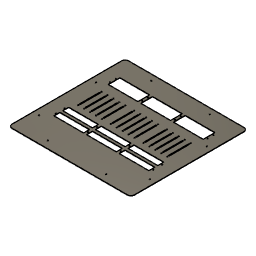
frontplate (Autodesk Fusion 360 design; units mm, degrees)
Autodesk Fusion 360 part; units mm, degrees
note: some values were not read from the file. Set by a fixed rule: which sketch regions a step uses.
sketch "Skizze1" plane through (0, 0, 0) normal (0, 1, 0) x (1, 0, 0)
  line L0 (198, -200) -> (-198, -200)
  line L1 (-210, -188) -> (-210, 188)
  line L2 (-198, 200) -> (198, 200)
  line L3 (210, 188) -> (210, -188)
  line L4 (210, -200) -> (-210, 200) construction
  line L5 (-210, -200) -> (210, 200) construction
  arc A0 (-198, 200) -> (-210, 188) centre (-198, 188) ccw
  arc A1 (210, 188) -> (198, 200) centre (198, 188) ccw
  arc A2 (198, -200) -> (210, -188) centre (198, -188) ccw
  arc A3 (-210, -188) -> (-198, -200) centre (-198, -188) ccw
  dimension "d1" = 420
  dimension "d2" = 400
  dimension "d3" = 12
  constraint perpendicular L0 L1
  constraint parallel L0 L2
  constraint parallel L1 L3
  constraint horizontal L0
  constraint coincident L4 origin
  constraint coincident L5 origin
  constraint coincident L4.end L1
  constraint coincident L4.end L2
  constraint tangent L1 A0
  constraint tangent L2 A0
  constraint coincident L5.end L2
  constraint coincident L5.end L3
  constraint tangent L2 A1
  constraint tangent L3 A1
  constraint equal A0 A1
  constraint coincident L4.start L3
  constraint coincident L4.start L0
  constraint tangent L3 A2
  constraint tangent L0 A2
  constraint equal A0 A2
  constraint coincident L5.start L1
  constraint coincident L5.start L0
  constraint tangent L1 A3
  constraint tangent L0 A3
  constraint equal A0 A3
  measures "d1" distance of L4.end L5.end
  measures "d2" distance of L5.start L4.end
  measures "d3" radius of A0
extrude "Fläche1" add sketch "Skizze1" along normal blind 1.5
sketch "Skizze2" plane through (0, 1.5, 0) normal (0, 1, 0) x (-1, 0, 0)
  arc A0 (198, -200) -> (210, -188) centre (198, -188) ccw
  line L0 (210, -188) -> (210, 188)
  arc A1 (210, 188) -> (198, 200) centre (198, 188) ccw
  line L1 (198, 200) -> (-198, 200)
  arc A2 (-198, 200) -> (-210, 188) centre (-198, 188) ccw
  line L2 (-210, 188) -> (-210, -188)
  arc A3 (-210, -188) -> (-198, -200) centre (-198, -188) ccw
  line L3 (-198, -200) -> (198, -200)
  circle A4 centre (-91.6, -62) radius 1.6
  line L4 (0, -62) -> (0, -57)
  line L5 (-130.9, -57) -> (-133.9, -57)
  line L6 (0, -200) -> (0, 200)
  line L7 (-110.5, 13) -> (-110.5, -57)
  circle A5 centre (-71.2, -62) radius 1.6
  line L8 (-110.5, -57) -> (-113.5, -57)
  line L9 (1.5, 13) -> (1.5, -57)
  line L10 (-69.7, 13) -> (-69.7, -57)
  circle A6 centre (-20.4, -62) radius 1.6
  circle A7 centre (0, -62) radius 1.6
  line L11 (-42.3, -57) -> (-42.3, 13)
  line L12 (-1.5, -57) -> (-1.5, 13)
  line L13 (-21.9, -57) -> (-21.9, 13)
  line L14 (-113.5, -57) -> (-113.5, 13)
  line L15 (-151.3, 13) -> (-151.3, -57)
  line L16 (-18.9, 13) -> (-18.9, -57)
  line L17 (-39.3, -57) -> (-42.3, -57)
  line L18 (-151.3, -57) -> (-154.3, -57)
  circle A8 centre (-40.8, -62) radius 1.6
  line L19 (210, -188) -> (210, 188)
  circle A9 centre (-132.4, -62) radius 1.6
  line L20 (-198, -200) -> (198, -200)
  line L21 (-130.9, 13) -> (-130.9, -57)
  line L22 (-18.9, -57) -> (-21.9, -57)
  line L23 (-210, 188) -> (-210, -188)
  circle A10 centre (-112, -62) radius 1.6
  line L24 (-39.3, 13) -> (-39.3, -57)
  line L25 (0, -57) -> (0, -62)
  line L26 (-10.2, 70.9) -> (10.2, 91.3) construction
  line L27 (72.7, 13) -> (72.7, -57)
  circle A11 centre (-168, -105) radius 1.6
  line L28 (154.3, 13) -> (154.3, -57)
  line L29 (-10.2, -135) -> (-30.6, -95) construction
  line L30 (-10.2, 40.5) -> (-30.6, 60.9) construction
  line L31 (72.7, -57) -> (69.7, -57)
  line L32 (154.3, -57) -> (151.3, -57)
  line L33 (133.9, -57) -> (130.9, -57)
  line L34 (-8.6, -135) -> (-8.6, -97)
  circle A12 centre (-20.4, 18) radius 1.6
  line L35 (198, 200) -> (-198, 200)
  line L36 (81.4, -135) -> (101.8, -95) construction
  line L37 (69.7, -57) -> (69.7, 13)
  line L38 (-51.8, -97) -> (-51.8, -135)
  line L39 (113.5, -57) -> (110.5, -57)
  line L40 (10.2, -95) -> (-10.2, -95)
  line L41 (-101.8, -135) -> (-81.4, -135)
  line L42 (0, 18) -> (0, 13)
  line L43 (113.5, 13) -> (113.5, -57)
  line L44 (-81.4, -135) -> (-61, -95) construction
  line L45 (-30.6, 60.9) -> (-30.6, 40.5)
  line L46 (-122.2, -135) -> (-101.8, -95) construction
  circle A13 centre (56, -105) radius 1.6
  circle A14 centre (40.8, -62) radius 1.6
  line L47 (10.2, 70.9) -> (-10.2, 91.3) construction
  line L48 (101.8, -135) -> (81.4, -95) construction
  line L49 (42.3, 13) -> (42.3, -57)
  circle A15 centre (112, -62) radius 1.6
  line L50 (-163, -95) -> (-163, -135)
  line L51 (-31.4, 84) -> (-31.4, 66)
  line L52 (-8.6, 66) -> (-8.6, 84)
  line L53 (-10.2, 70.9) -> (-30.6, 91.3) construction
  line L54 (-101.8, -135) -> (-101.8, -95)
  line L55 (-122.2, -95) -> (-142.6, -95)
  circle A16 centre (20.4, -62) radius 1.6
  line L56 (11.8, -135) -> (11.8, -97)
  line L57 (-30.6, -135) -> (-51, -95) construction
  line L58 (-81.4, -95) -> (-101.8, -95)
  line L59 (29.8, -97) -> (29.8, -135)
  line L60 (-51, -125) -> (-61, -125)
  line L61 (-51, -135) -> (-30.6, -95) construction
  line L62 (61, -95) -> (61, -135)
  line L63 (-142.6, -95) -> (-163, -95)
  line L64 (-10.2, 70.9) -> (-10.2, 91.3)
  line L65 (-81.4, -135) -> (-81.4, -95)
  line L66 (30.6, -135) -> (10.2, -95) construction
  line L67 (-10.2, 60.9) -> (-30.6, 60.9)
  line L68 (81.4, 40.5) -> (81.4, 60.9)
  line L69 (-101.8, -135) -> (-122.2, -95) construction
  line L70 (-30.6, 70.9) -> (-10.2, 70.9)
  line L71 (-142.6, -135) -> (-142.6, -95)
  line L72 (-101.8, -135) -> (-81.4, -95) construction
  line L73 (30.6, -95) -> (30.6, -135)
  line L74 (-163, -135) -> (-142.6, -135)
  line L75 (133.9, 13) -> (133.9, -57)
  line L76 (-11, -97) -> (-11, -135)
  line L77 (10.2, -135) -> (30.6, -135)
  circle A17 centre (-56, -125) radius 1.6
  line L78 (81.4, -135) -> (101.8, -135)
  circle A18 centre (152.8, -62) radius 1.6
  circle A19 centre (71.2, -62) radius 1.6
  line L79 (61, 40.5) -> (81.4, 40.5)
  line L80 (-81.4, -135) -> (-61, -135)
  line L81 (-122.2, -135) -> (-101.8, -135)
  line L82 (-122.2, -135) -> (-122.2, -95)
  line L83 (-122.2, -95) -> (-122.2, -135)
  line L84 (-10.2, -135) -> (-10.2, -95)
  line L85 (-10.2, 40.5) -> (10.2, 60.9) construction
  line L86 (-10.2, 91.3) -> (-10.2, 70.9)
  line L87 (-61, -135) -> (-61, -95)
  line L88 (18.9, -57) -> (18.9, 13)
  line L89 (10.2, 60.9) -> (-10.2, 60.9)
  line L90 (-30.6, 70.9) -> (-10.2, 91.3) construction
  circle A20 centre (56, -125) radius 1.6
  line L91 (30.6, -135) -> (30.6, -95)
  circle A21 centre (0, 18) radius 1.6
  line L92 (42.3, -57) -> (39.3, -57)
  line L93 (30.6, -135) -> (51, -135)
  line L94 (-30.6, -135) -> (-10.2, -95) construction
  line L95 (-122.2, -135) -> (-142.6, -95) construction
  circle A22 centre (91.6, -62) radius 1.6
  line L96 (-30.6, 91.3) -> (-30.6, 70.9)
  line L97 (21.9, -57) -> (18.9, -57)
  line L98 (51, 40.5) -> (51, 60.9)
  line L99 (51, -135) -> (30.6, -95) construction
  line L100 (-51, -95) -> (-51, -135)
  line L101 (-49.4, -135) -> (-49.4, -97)
  line L102 (69.7, 13) -> (72.7, 13)
  line L103 (61, -105) -> (51, -105)
  line L104 (151.3, -57) -> (151.3, 13)
  line L105 (-10.2, -135) -> (10.2, -95) construction
  line L106 (-61, -135) -> (-81.4, -95) construction
  line L107 (39.3, -57) -> (39.3, 13)
  line L108 (101.8, 91.3) -> (81.4, 91.3)
  line L109 (-122.2, 70.9) -> (-122.2, 91.3)
  line L110 (-81.4, -135) -> (-101.8, -95) construction
  line L111 (-61, -95) -> (-81.4, -95)
  line L112 (61, -135) -> (81.4, -135)
  line L113 (-21.9, 13) -> (-18.9, 13)
  line L114 (-101.8, -95) -> (-101.8, -135)
  line L115 (-122.2, 70.9) -> (-101.8, 70.9)
  circle A23 centre (20.4, 18) radius 1.6
  line L116 (-10.2, 40.5) -> (-10.2, 60.9)
  line L117 (110.5, -57) -> (110.5, 13)
  line L118 (-30.6, 70.9) -> (-30.6, 91.3)
  line L119 (-11, 56) -> (-11, 38)
  line L120 (130.9, -57) -> (130.9, 13)
  line L121 (122.2, 91.3) -> (101.8, 91.3)
  line L122 (61, -125) -> (51, -125)
  line L123 (-142.6, -135) -> (-122.2, -95) construction
  line L124 (-101.8, 70.9) -> (-81.4, 70.9)
  line L125 (101.8, -95) -> (81.4, -95)
  line L126 (-30.6, -135) -> (-10.2, -135)
  line L127 (-122.2, 40.5) -> (-101.8, 40.5)
  line L128 (51, 91.3) -> (30.6, 91.3)
  line L129 (10.2, 40.5) -> (10.2, 60.9)
  line L130 (30.6, 60.9) -> (30.6, 40.5)
  line L131 (-51, -135) -> (-30.6, -135)
  line L132 (142.6, -135) -> (163, -135)
  line L133 (-10.2, 60.9) -> (-10.2, 40.5)
  line L134 (-122.2, 91.3) -> (-142.6, 91.3)
  line L135 (-10.2, 40.5) -> (10.2, 40.5)
  line L136 (-101.8, 40.5) -> (-81.4, 40.5)
  line L137 (-81.4, 40.5) -> (-101.8, 60.9) construction
  line L138 (61, 60.9) -> (61, 40.5)
  line L139 (-81.4, 91.3) -> (-101.8, 91.3)
  line L140 (30.6, 40.5) -> (10.2, 60.9) construction
  line L141 (11.8, 38) -> (11.8, 56)
  line L142 (142.6, -135) -> (122.2, -95) construction
  line L143 (-30.6, 40.5) -> (-10.2, 40.5)
  circle A24 centre (71.2, 18) radius 1.6
  circle A25 centre (166.5, -105) radius 1.6
  line L144 (-101.8, 60.9) -> (-122.2, 60.9)
  line L145 (-122.2, 70.9) -> (-101.8, 91.3) construction
  line L146 (101.8, -135) -> (101.8, -95)
  line L147 (-113.5, 13) -> (-110.5, 13)
  line L148 (-101.8, 91.3) -> (-122.2, 91.3)
  line L149 (-122.2, 60.9) -> (-122.2, 40.5)
  circle A26 centre (-56, 81.1) radius 1.6
  line L150 (81.4, 60.9) -> (61, 60.9)
  line L151 (61, 40.5) -> (81.4, 60.9) construction
  line L152 (-51.8, 56) -> (-51.8, 38)
  line L153 (163, -105) -> (166.5, -105)
  line L154 (-30.6, -95) -> (-30.6, -135)
  line L155 (30.6, 60.9) -> (10.2, 60.9)
  line L156 (-122.2, 91.3) -> (-122.2, 70.9)
  line L157 (10.2, -135) -> (-10.2, -95) construction
  line L158 (10.2, 40.5) -> (30.6, 60.9) construction
  line L159 (-11, 84) -> (-11, 66)
  line L160 (142.6, -95) -> (122.2, -95)
  line L161 (-101.8, 70.9) -> (-101.8, 91.3)
  line L162 (10.2, 60.9) -> (10.2, 40.5)
  line L163 (-51, 81.1) -> (-61, 81.1)
  line L164 (30.6, -95) -> (10.2, -95)
  line L165 (-142.6, 91.3) -> (-163, 91.3)
  line L166 (122.2, -95) -> (122.2, -135)
  line L167 (-122.2, 40.5) -> (-101.8, 60.9) construction
  line L168 (10.2, 40.5) -> (30.6, 40.5)
  line L169 (122.2, -135) -> (142.6, -95) construction
  line L170 (-93.1, 13) -> (-90.1, 13)
  circle A27 centre (40.8, 18) radius 1.6
  line L171 (163, -125) -> (166.5, -125)
  line L172 (122.2, -135) -> (101.8, -95) construction
  line L173 (-51, 50.7) -> (-61, 50.7)
  line L174 (-72.7, 13) -> (-69.7, 13)
  circle A28 centre (166.5, -125) radius 1.6
  arc A29 (-198, 200) -> (-210, 188) centre (-198, 188) ccw
  line L175 (-81.4, 70.9) -> (-61, 91.3) construction
  line L176 (-81.4, 40.5) -> (-61, 40.5)
  line L177 (122.2, -135) -> (142.6, -135)
  line L178 (163, -95) -> (142.6, -95)
  line L179 (-30.6, 60.9) -> (-51, 60.9)
  line L180 (-42.3, 13) -> (-39.3, 13)
  line L181 (-30.6, 40.5) -> (-51, 60.9) construction
  line L182 (101.8, -135) -> (122.2, -135)
  line L183 (101.8, -95) -> (101.8, -135)
  line L184 (142.6, -135) -> (163, -95) construction
  line L185 (-51, 40.5) -> (-30.6, 40.5)
  line L186 (61, 50.7) -> (51, 50.7)
  line L187 (163, -135) -> (142.6, -95) construction
  line L188 (-81.4, 70.9) -> (-101.8, 91.3) construction
  line L189 (30.6, 40.5) -> (30.6, 60.9)
  line L190 (-81.4, 70.9) -> (-61, 70.9)
  line L191 (-61, 70.9) -> (-81.4, 91.3) construction
  line L192 (163, 91.3) -> (142.6, 91.3)
  line L193 (-101.8, 70.9) -> (-81.4, 91.3) construction
  line L194 (-8.6, 38) -> (-8.6, 56)
  line L195 (81.4, -135) -> (81.4, -95)
  line L196 (-163, -135) -> (-142.6, -95) construction
  line L197 (-29, 38) -> (-29, 56)
  line L198 (-29, -135) -> (-29, -97)
  circle A30 centre (132.4, -62) radius 1.6
  line L199 (93.1, 13) -> (93.1, -57)
  line L200 (-1.5, 13) -> (1.5, 13)
  line L201 (-30.6, 40.5) -> (-30.6, 60.9)
  line L202 (-10.2, -135) -> (10.2, -135)
  line L203 (10.2, 40.5) -> (-10.2, 60.9) construction
  line L204 (-101.8, -95) -> (-122.2, -95)
  circle A31 centre (56, 50.7) radius 1.6
  line L205 (81.4, 60.9) -> (81.4, 40.5)
  line L206 (51, -95) -> (30.6, -95)
  line L207 (-51, -105) -> (-61, -105)
  line L208 (-142.6, -95) -> (-142.6, -135)
  line L209 (30.6, 40.5) -> (51, 40.5)
  line L210 (81.4, -95) -> (61, -95)
  line L211 (21.9, 13) -> (21.9, -57)
  line L212 (-31.4, 56) -> (-31.4, 38)
  line L213 (-101.8, 40.5) -> (-101.8, 60.9)
  line L214 (90.1, -57) -> (90.1, 13)
  line L215 (142.6, 91.3) -> (122.2, 91.3)
  line L216 (-101.8, 91.3) -> (-101.8, 70.9)
  line L217 (30.6, -135) -> (51, -95) construction
  line L218 (81.4, 40.5) -> (61, 60.9) construction
  line L219 (93.1, -57) -> (90.1, -57)
  line L220 (-142.6, -135) -> (-163, -95) construction
  circle A32 centre (-168, -125) radius 1.6
  line L221 (-101.8, 60.9) -> (-101.8, 40.5)
  line L222 (10.2, 91.3) -> (-10.2, 91.3)
  line L223 (-30.6, -95) -> (-51, -95)
  line L224 (30.6, 91.3) -> (10.2, 91.3)
  line L225 (61, -135) -> (81.4, -95) construction
  line L226 (51, 60.9) -> (30.6, 60.9)
  line L227 (81.4, -135) -> (61, -95) construction
  line L228 (-30.6, -135) -> (-30.6, -95)
  line L229 (-81.4, -95) -> (-81.4, -135)
  line L230 (-101.8, 40.5) -> (-81.4, 60.9) construction
  line L231 (-142.6, -135) -> (-122.2, -135)
  line L232 (51, -135) -> (51, -95)
  line L233 (30.6, 40.5) -> (51, 60.9) construction
  line L234 (81.4, 91.3) -> (61, 91.3)
  circle A33 centre (-112, 18) radius 1.6
  line L235 (-81.4, 60.9) -> (-101.8, 60.9)
  line L236 (29.8, 56) -> (29.8, 38)
  line L237 (-10.2, 91.3) -> (-30.6, 91.3)
  line L238 (9.4, 56) -> (9.4, 38)
  line L239 (122.2, -135) -> (122.2, -95)
  line L240 (10.2, -135) -> (30.6, -95) construction
  line L241 (-31.4, -97) -> (-31.4, -135)
  line L242 (-101.8, 70.9) -> (-122.2, 91.3) construction
  line L243 (9.4, -97) -> (9.4, -135)
  line L244 (-10.2, -95) -> (-10.2, -135)
  line L245 (10.2, -95) -> (10.2, -135)
  circle A34 centre (-91.6, 18) radius 1.6
  line L246 (81.4, -95) -> (81.4, -135)
  line L247 (-29, 66) -> (-29, 84)
  line L248 (-10.2, -95) -> (-30.6, -95)
  line L249 (18.9, 13) -> (21.9, 13)
  line L250 (-101.8, 40.5) -> (-122.2, 60.9) construction
  line L251 (51, 40.5) -> (30.6, 60.9) construction
  line L252 (-69.8, -135) -> (-69.8, -97)
  line L253 (-10.2, 70.9) -> (10.2, 70.9)
  line L254 (-122.2, 40.5) -> (-122.2, 60.9)
  circle A35 centre (-56, -105) radius 1.6
  line L255 (10.2, -135) -> (10.2, -95)
  line L256 (39.3, 13) -> (42.3, 13)
  line L257 (-30.6, 40.5) -> (-10.2, 60.9) construction
  line L258 (-51.8, 84) -> (-51.8, 66)
  line L259 (-142.6, 70.9) -> (-163, 91.3) construction
  line L260 (81.4, 91.3) -> (81.4, 70.9)
  line L261 (-69.8, 66) -> (-69.8, 84)
  line L262 (11.8, 66) -> (11.8, 84)
  line L263 (-163, 60.9) -> (-163, 40.5)
  line L264 (81.4, 40.5) -> (101.8, 60.9) construction
  line L265 (-51, 60.9) -> (-51, 40.5)
  line L266 (-154.3, 13) -> (-151.3, 13)
  line L267 (29.8, 84) -> (29.8, 66)
  arc A36 (210, 188) -> (198, 200) centre (198, 188) ccw
  line L268 (61, 70.9) -> (81.4, 70.9)
  line L269 (51, 70.9) -> (30.6, 91.3) construction
  line L270 (-142.6, 40.5) -> (-163, 60.9) construction
  line L271 (-163, 50.7) -> (-168, 50.7)
  line L272 (-142.6, 70.9) -> (-122.2, 70.9)
  line L273 (122.2, 40.5) -> (122.2, 60.9)
  line L274 (-81.4, 40.5) -> (-61, 60.9) construction
  line L275 (-51, 91.3) -> (-51, 70.9)
  line L276 (-51, 70.9) -> (-30.6, 91.3) construction
  line L277 (10.2, 91.3) -> (10.2, 70.9)
  line L278 (-51, 70.9) -> (-30.6, 70.9)
  line L279 (101.8, 60.9) -> (81.4, 60.9)
  line L280 (-142.6, 91.3) -> (-142.6, 70.9)
  line L281 (-61, 60.9) -> (-81.4, 60.9)
  line L282 (101.8, 40.5) -> (122.2, 60.9) construction
  line L283 (81.4, 70.9) -> (81.4, 91.3)
  line L284 (110.5, 13) -> (113.5, 13)
  line L285 (122.2, 60.9) -> (101.8, 60.9)
  line L286 (-49.4, 38) -> (-49.4, 56)
  line L287 (-142.6, 70.9) -> (-142.6, 91.3)
  line L288 (-163, 81.1) -> (-168, 81.1)
  line L289 (101.8, 40.5) -> (122.2, 40.5)
  line L290 (61, 91.3) -> (61, 70.9)
  line L291 (122.2, 70.9) -> (122.2, 91.3)
  line L292 (122.2, 70.9) -> (101.8, 91.3) construction
  line L293 (101.8, 70.9) -> (122.2, 91.3) construction
  line L294 (-81.4, 60.9) -> (-81.4, 40.5)
  line L295 (-61, 40.5) -> (-81.4, 60.9) construction
  line L296 (-133.9, 13) -> (-130.9, 13)
  line L297 (10.2, 70.9) -> (30.6, 91.3) construction
  line L298 (163, 81.1) -> (166.5, 81.1)
  circle A37 centre (-56, 50.7) radius 1.6
  circle A38 centre (-168, 50.7) radius 1.6
  line L299 (9.4, 84) -> (9.4, 66)
  line L300 (-61, 91.3) -> (-81.4, 91.3)
  circle A39 centre (112, 18) radius 1.6
  line L301 (-81.4, 40.5) -> (-81.4, 60.9)
  circle A40 centre (-71.2, 18) radius 1.6
  line L302 (-142.6, 60.9) -> (-163, 60.9)
  circle A41 centre (-152.8, 18) radius 1.6
  circle A42 centre (91.6, 18) radius 1.6
  line L303 (51, 70.9) -> (51, 91.3)
  line L304 (-122.2, 70.9) -> (-142.6, 91.3) construction
  line L305 (-122.2, 60.9) -> (-142.6, 60.9)
  line L306 (-163, 40.5) -> (-142.6, 60.9) construction
  line L307 (90.1, 13) -> (93.1, 13)
  line L308 (122.2, 40.5) -> (101.8, 60.9) construction
  line L309 (101.8, 70.9) -> (122.2, 70.9)
  line L310 (-142.6, 40.5) -> (-122.2, 40.5)
  line L311 (30.6, 70.9) -> (10.2, 91.3) construction
  line L312 (10.2, 70.9) -> (30.6, 70.9)
  line L313 (-163, 70.9) -> (-142.6, 70.9)
  line L314 (30.6, 91.3) -> (30.6, 70.9)
  line L315 (142.6, -135) -> (142.6, -95)
  line L316 (163, -135) -> (163, -95)
  line L317 (-30.6, 91.3) -> (-51, 91.3)
  circle A43 centre (-40.8, 18) radius 1.6
  line L318 (-61, 70.9) -> (-61, 91.3)
  line L319 (30.6, 70.9) -> (51, 70.9)
  line L320 (61, 81.1) -> (51, 81.1)
  line L321 (-163, 70.9) -> (-142.6, 91.3) construction
  line L322 (-81.4, 70.9) -> (-81.4, 91.3)
  line L323 (-49.4, 66) -> (-49.4, 84)
  line L324 (-142.6, 70.9) -> (-122.2, 91.3) construction
  line L325 (142.6, -95) -> (142.6, -135)
  line L326 (101.8, -135) -> (122.2, -95) construction
  line L327 (30.6, 70.9) -> (51, 91.3) construction
  arc A44 (-210, -188) -> (-198, -200) centre (-198, -188) ccw
  arc A45 (198, -200) -> (210, -188) centre (198, -188) ccw
  line L328 (61, 70.9) -> (81.4, 91.3) construction
  circle A46 centre (-168, 81.1) radius 1.6
  line L329 (122.2, -95) -> (101.8, -95)
  line L330 (-30.6, 70.9) -> (-51, 91.3) construction
  line L331 (-122.2, 40.5) -> (-142.6, 60.9) construction
  line L332 (-69.8, 38) -> (-69.8, 56)
  line L333 (10.2, 70.9) -> (10.2, 91.3)
  line L334 (-163, 91.3) -> (-163, 70.9)
  line L335 (-81.4, 91.3) -> (-81.4, 70.9)
  line L336 (-61, 40.5) -> (-61, 60.9)
  line L337 (30.6, 70.9) -> (30.6, 91.3)
  circle A47 centre (-132.4, 18) radius 1.6
  line L338 (-142.6, 40.5) -> (-122.2, 60.9) construction
  line L339 (-51, 40.5) -> (-30.6, 60.9) construction
  circle A48 centre (56, 81.1) radius 1.6
  line L340 (81.4, 70.9) -> (61, 91.3) construction
  line L341 (-163, 40.5) -> (-142.6, 40.5)
  line L342 (0, -62) -> (0, -57)
  line L343 (-90.1, -57) -> (-93.1, -57)
  line L344 (-93.1, -57) -> (-93.1, 13)
  line L345 (1.5, -57) -> (-1.5, -57)
  line L346 (-133.9, -57) -> (-133.9, 13)
  circle A49 centre (-152.8, -62) radius 1.6
  line L347 (-72.7, -57) -> (-72.7, 13)
  line L348 (-154.3, -57) -> (-154.3, 13)
  line L349 (-69.7, -57) -> (-72.7, -57)
  line L350 (-90.1, 13) -> (-90.1, -57)
  circle A50 centre (166.5, 50.7) radius 1.6
  line L351 (163, 40.5) -> (163, 60.9)
  line L352 (151.3, 13) -> (154.3, 13)
  line L353 (163, 70.9) -> (142.6, 91.3) construction
  line L354 (163, 70.9) -> (163, 91.3)
  line L355 (142.6, 60.9) -> (122.2, 60.9)
  line L356 (163, 50.7) -> (166.5, 50.7)
  line L357 (142.6, 40.5) -> (163, 40.5)
  line L358 (122.2, 40.5) -> (142.6, 40.5)
  line L359 (130.9, 13) -> (133.9, 13)
  line L360 (142.6, 40.5) -> (122.2, 60.9) construction
  circle A51 centre (166.5, 81.1) radius 1.6
  line L361 (142.6, 70.9) -> (163, 91.3) construction
  circle A52 centre (152.8, 18) radius 1.6
  line L362 (163, 60.9) -> (142.6, 60.9)
  line L363 (142.6, 40.5) -> (163, 60.9) construction
  line L364 (142.6, 40.5) -> (142.6, 60.9)
  line L365 (142.6, 70.9) -> (122.2, 91.3) construction
  line L366 (81.4, 70.9) -> (101.8, 70.9)
  line L367 (101.8, 40.5) -> (81.4, 60.9) construction
  line L368 (122.2, 60.9) -> (122.2, 40.5)
  line L369 (-142.6, 40.5) -> (-142.6, 60.9)
  line L370 (-142.6, 60.9) -> (-142.6, 40.5)
  line L371 (122.2, 91.3) -> (122.2, 70.9)
  line L372 (101.8, 60.9) -> (101.8, 40.5)
  line L373 (101.8, 70.9) -> (81.4, 91.3) construction
  line L374 (81.4, 70.9) -> (101.8, 91.3) construction
  line L375 (101.8, 91.3) -> (101.8, 70.9)
  line L376 (81.4, 40.5) -> (101.8, 40.5)
  line L377 (101.8, 70.9) -> (101.8, 91.3)
  line L378 (101.8, 40.5) -> (101.8, 60.9)
  line L379 (142.6, 70.9) -> (163, 70.9)
  line L380 (142.6, 91.3) -> (142.6, 70.9)
  line L381 (122.2, 70.9) -> (142.6, 70.9)
  line L382 (142.6, 60.9) -> (142.6, 40.5)
  line L383 (163, 40.5) -> (142.6, 60.9) construction
  circle A53 centre (132.4, 18) radius 1.6
  line L384 (142.6, 70.9) -> (142.6, 91.3)
  line L385 (122.2, 40.5) -> (142.6, 60.9) construction
  line L386 (122.2, 70.9) -> (142.6, 91.3) construction
  point P0 (-112, 81.1)
  point P1 (-112, 50.7)
  point P2 (112, 81.1)
  point P3 (-132.4, -115)
  point P4 (56, 50.7)
  point P5 (42.2, 66)
  point P6 (123.8, 38)
  point P7 (56, 81.1)
  point P8 (80.6, 56)
  point P9 (141.8, -135)
  point P10 (101, -97)
  point P11 (80.6, 66)
  point P12 (0, 13)
  point P13 (-181.8, 66)
  point P14 (121.4, 84)
  point P15 (121.4, 66)
  point P16 (-143.4, 56)
  point P17 (80.6, 38)
  point P18 (83, -97)
  point P19 (101, 38)
  point P20 (-143.4, 66)
  point P21 (80.6, -135)
  point P22 (83, 56)
  point P23 (141.8, 38)
  point P24 (-82.2, -135)
  point P25 (-100.2, 38)
  point P26 (123.8, 84)
  point P27 (62.6, 38)
  point P28 (103.4, 38)
  point P29 (62.6, -97)
  point P30 (101, 66)
  point P31 (141.8, 56)
  point P32 (60.2, 84)
  point P33 (60.2, -97)
  point P34 (121.4, 56)
  point P35 (91.6, 81.1)
  point P36 (-141, 84)
  point P37 (-181.8, -135)
  point P38 (-123, -97)
  point P39 (-123, -135)
  point P40 (-82.2, -97)
  point P41 (-161.4, -135)
  point P42 (-120.6, -97)
  point P43 (-102.6, -97)
  point P44 (-163.8, 56)
  point P45 (-120.6, -135)
  point P46 (-100.2, -135)
  point P47 (-100.2, -97)
  point P48 (-102.6, -135)
  point P49 (-181.8, -97)
  point P50 (20.4, -115)
  point P51 (20.4, 81.1)
  point P52 (-91.6, 81.1)
  point P53 (-100.2, 56)
  point P54 (-181.8, 56)
  point P55 (-163.8, 38)
  point P56 (-141, -135)
  point P57 (-120.6, 84)
  point P58 (-161.4, 84)
  point P59 (-163.8, -135)
  point P60 (-82.2, 66)
  point P61 (-161.4, -97)
  point P62 (-163.8, 84)
  point P63 (-120.6, 38)
  point P64 (-82.2, 56)
  point P65 (-163.8, -97)
  point P66 (-141, 38)
  point P67 (91.6, 50.7)
  point P68 (132.4, -115)
  point P69 (152.8, -115)
  point P70 (152.8, 50.7)
  point P71 (170, -200)
  point P72 (-132.4, 81.1)
  point P73 (101, 84)
  point P74 (80.6, 84)
  point P75 (62.6, 56)
  point P76 (42.2, 38)
  point P77 (101, 56)
  point P78 (121.4, 38)
  point P79 (80.6, -97)
  point P80 (60.2, 66)
  point P81 (62.6, 66)
  point P82 (83, 66)
  point P83 (103.4, 56)
  point P84 (103.4, 66)
  point P85 (42.2, 84)
  point P86 (141.8, 84)
  point P87 (-152.8, 50.7)
  point P88 (-91.6, 50.7)
  point P89 (83, -135)
  point P90 (83, 38)
  point P91 (123.8, 56)
  point P92 (0, -57)
  point P93 (62.6, 84)
  point P94 (42.2, 56)
  point P95 (103.4, 84)
  point P96 (60.2, -135)
  point P97 (60.2, 38)
  point P98 (-102.6, 38)
  point P99 (-102.6, 56)
  point P100 (-181.8, 84)
  point P101 (-82.2, 84)
  point P102 (-161.4, 66)
  point P103 (-120.6, 56)
  point P104 (-143.4, 84)
  point P105 (-120.6, 66)
  point P106 (-123, 56)
  point P107 (-161.4, 38)
  point P108 (-163.8, 66)
  point P109 (-143.4, -97)
  point P110 (-161.4, 56)
  point P111 (-123, 66)
  point P112 (40.8, -115)
  point P113 (71.2, 81.1)
  point P114 (56, -125)
  point P115 (-56, -125)
  point P116 (-56, -105)
  point P117 (121.4, -135)
  point P118 (123.8, -97)
  point P119 (42.2, -135)
  point P120 (42.2, -97)
  point P121 (103.4, -97)
  point P122 (141.8, -97)
  point P123 (121.4, -97)
  point P124 (62.6, -135)
  point P125 (60.2, 56)
  point P126 (83, 84)
  point P127 (103.4, -135)
  point P128 (101, -135)
  point P129 (123.8, -135)
  point P130 (141.8, 66)
  point P131 (0, -115)
  point P132 (20.4, 50.7)
  point P133 (-132.4, 50.7)
  point P134 (-152.8, 81.1)
  point P135 (-40.8, -115)
  point P136 (-40.8, 50.7)
  point P137 (-40.8, 81.1)
  point P138 (0, 81.1)
  point P139 (0, 50.7)
  point P140 (112, -115)
  point P141 (40.8, 50.7)
  point P142 (40.8, 81.1)
  point P143 (-71.2, 81.1)
  point P144 (-112, -115)
  point P145 (-152.8, -115)
  point P146 (-20.4, 50.7)
  point P147 (71.2, -115)
  point P148 (152.8, 81.1)
  point P149 (-71.2, 50.7)
  point P150 (-123, 84)
  point P151 (-141, 56)
  point P152 (-141, -97)
  point P153 (-141, 66)
  point P154 (-123, 38)
  point P155 (-102.6, 66)
  point P156 (-143.4, -135)
  point P157 (0, -125)
  point P158 (-100.2, 84)
  point P159 (-102.6, 84)
  point P160 (0, -105)
  point P161 (-82.2, 38)
  point P162 (-143.4, 38)
  point P163 (-181.8, 38)
  point P164 (-56, 50.7)
  point P165 (-56, 81.1)
  point P166 (-20.4, -115)
  point P167 (-20.4, 81.1)
  point P168 (56, -105)
  point P169 (91.6, -115)
  point P170 (-91.6, -115)
  point P171 (-71.2, -115)
  point P172 (112, 50.7)
  point P173 (132.4, 81.1)
  point P174 (71.2, 50.7)
  point P175 (132.4, 50.7)
  dimension "d7" = 40.8
  dimension "d8" = 0
  dimension "d11" = 112
  dimension "d12" = 0
  dimension "d13" = 70
  dimension "d14" = 3
  dimension "d15" = 20.4
  dimension "d16" = 10
  dimension "d17" = 27.5
  dimension "d18" = 40
  dimension "d19" = 38
  dimension "d20" = 65
  dimension "d21" = 10
  dimension "d22" = 20
  dimension "d23" = 3.2
  dimension "d24" = 3.2
  dimension "d25" = 3.2
  dimension "d26" = 3.2
  dimension "d27" = 3.2
  dimension "d28" = 3.2
  dimension "d29" = 3.2
  dimension "d30" = 3.2
  dimension "d31" = 5
  dimension "d32" = 3.5
  dimension "d33" = 10
  dimension "d34" = 3.5
  dimension "d35" = 3.2
  dimension "d36" = 10
  dimension "d37" = 3.5
  dimension "d38" = 3.2
  dimension "d39" = 10
  dimension "d40" = 10
  dimension "d41" = 3.2
  dimension "d42" = 3.2
  dimension "d43" = 10
  dimension "d44" = 10
  dimension "d45" = 3.2
  dimension "d46" = 3.2
  dimension "d47" = 3.2
  dimension "d48" = 3.2
  dimension "d49" = 5
  dimension "d50" = 5
  dimension "d51" = 10
  dimension "d52" = 10
  dimension "d53" = 3.2
  dimension "d54" = 5
  dimension "d55" = 5
  constraint midpoint L6.start L20
  constraint midpoint L6.end L35
  constraint horizontal L345
  constraint vertical L12
  constraint horizontal L200
  constraint vertical L9
  constraint symmetric L6 L9 L12
  constraint perpendicular L129 L135
  constraint parallel L89 L135
  constraint parallel L129 L133
  constraint horizontal L135
  constraint coincident P139 L85
  constraint coincident P139 L203
  constraint coincident P139 L6
  constraint perpendicular L253 L333
  constraint parallel L222 L253
  constraint parallel L86 L333
  constraint horizontal L253
  constraint coincident P138 L26
  constraint coincident P138 L47
  constraint coincident P138 L6
  constraint perpendicular L202 L255
  constraint parallel L40 L202
  constraint parallel L244 L255
  constraint horizontal L202
  constraint coincident P131 L105
  constraint coincident P131 L157
  constraint coincident P131 L6
  constraint equal L135 L253
  constraint equal L135 L202
  constraint equal L129 L135
  constraint equal L253 L333
  constraint coincident L42.start L6
  constraint coincident L4.start L6
  constraint equal A7 A21
  constraint coincident P157 L6
  constraint coincident P160 L6
  constraint midpoint L320.start L290
  constraint midpoint L320.end L303
  constraint midpoint P7 L320
  constraint midpoint L186.start L138
  constraint midpoint L186.end L98
  constraint midpoint P4 L186
  constraint midpoint L173.start L265
  constraint midpoint L173.end L336
  constraint midpoint L163.start L275
  constraint midpoint L163.end L318
  constraint midpoint P164 L173
  constraint midpoint P165 L163
  constraint coincident P4 A31.centre
  constraint coincident P7 A48.centre
  constraint coincident P164 A37.centre
  constraint coincident P165 A26.centre
  constraint midpoint L356.start L351
  constraint perpendicular L351 L356
  constraint coincident A50.centre L356.end
  constraint midpoint L298.start L354
  constraint perpendicular L298 L354
  constraint coincident L298.end A51.centre
  constraint equal L298 L356
  constraint midpoint L288.start L334
  constraint perpendicular L288 L334
  constraint coincident L288.end A46.centre
  constraint midpoint L271.start L263
  constraint perpendicular L263 L271
  constraint coincident L271.end A38.centre
  constraint equal L271 L288
  constraint coincident L153.start L316
  constraint perpendicular L153 L316
  constraint coincident A25.centre L153.end
  constraint coincident L171.start L316
  constraint perpendicular L171 L316
  constraint coincident L171.end A28.centre
  constraint coincident L122.start L62
  constraint coincident L122.end L232
  constraint perpendicular L122 L232
  constraint coincident L103.start L62
  constraint coincident L103.end L232
  constraint perpendicular L103 L232
  constraint midpoint P168 L103
  constraint midpoint P114 L122
  constraint coincident P114 A20.centre
  constraint coincident P168 A13.centre
  constraint coincident L60.start L100
  constraint coincident L60.end L87
  constraint perpendicular L60 L87
  constraint coincident L207.start L100
  constraint coincident L207.end L87
  constraint perpendicular L87 L207
  constraint midpoint P115 L60
  constraint midpoint P116 L207
  constraint coincident P115 A17.centre
  constraint coincident P116 A35.centre
  constraint coincident L4.start A7.centre
  constraint midpoint P92 L345
  constraint midpoint P12 L200
  constraint coincident L42.start A21.centre
  constraint coincident P12 L42.end
  constraint coincident P92 L4.end
  measures "d13" distance of L9.end L9.start
  measures "d14" distance of L12.start L9.end
  measures "d15" distance of L77.start L29.start
  measures "d16" distance of L89 L253
  measures "d17" distance of L135 L200
  measures "d18" distance of L40 L202
  measures "d19" distance of L40 L345
  measures "d20" distance of L20 L202
  measures "d21" distance of P160 L40
  measures "d22" distance of P157 P160
  measures "d23" diameter of A31
  measures "d24" diameter of A48
  measures "d25" diameter of A37
  measures "d26" diameter of A26
  measures "d27" diameter of A50
  measures "d28" diameter of A51
  measures "d29" diameter of A46
  measures "d30" diameter of A38
  measures "d31" distance of L271.start L271.end
  measures "d32" distance of L356.start A50.centre
  measures "d33" distance of L178.start L153.start
  measures "d34" distance of L153.start A25.centre
  measures "d35" diameter of A25
  measures "d36" distance of L132.end L171.start
  measures "d37" distance of L171.end L171.start
  measures "d38" diameter of A28
  measures "d39" distance of L122.start L62.end
  measures "d40" distance of L62.start L103.start
  measures "d41" diameter of A20
  measures "d42" diameter of A13
  measures "d43" distance of L60.start L61.start
  measures "d44" distance of L207.start L57.end
  measures "d45" diameter of A17
  measures "d46" diameter of A35
  measures "d47" diameter of A32
  measures "d48" diameter of A11
  measures "d49" distance of A32.centre L50
  measures "d50" distance of A11.centre L50
  measures "d51" vertical distance of L50.start A11.centre
  measures "d52" vertical distance of L50.end A32.centre
  measures "d53" diameter of A7
  measures "d54" distance of P92 L4.start
  measures "d55" distance of P12 L42.start
extrude "Extrusion1" cut sketch "Skizze2" against normal blind 5 contours L6 L40 L84 L202 L244 | L6 L40 L202 L245 L255 | L4 L6 A7 L25 L342 | L4 L6 A7 L25 L342 | L73 L77 L91 L164 L245 L255 | L84 L126 L154 L228 L244 L248 | L6 L222 L253 L277 L333 | L6 L64 L86 L222 L253 | L73 L91 L93 L206 L232 | L100 L131 L154 L223 L228 | L224 L277 L312 L314 L333 L337 | L64 L70 L86 L96 L118 L237 | L6 L12 L200 L345 | L6 L9 L200 L345 | L6 L89 L129 L135 L162 | L6 L89 L116 L133 L135 | L128 L303 L314 L319 L337 | L96 L118 L275 L278 L317 | L129 L130 L155 L162 L168 L189 | L45 L67 L116 L133 L143 L201 | L6 L42 A21 | L6 L42 A21 | A13 L103 | A13 L103 | L98 L130 L189 L209 L226 | L45 L179 L185 L201 L265 | A20 L122 | A20 L122 | L207 A35 | L207 A35 | L62 L112 L195 L210 L246 | L60 A17 | L60 A17 | L65 L80 L87 L111 L229 | L78 L125 L146 L183 L195 L246 | L146 L166 L182 L183 L239 L329 | L41 L54 L58 L65 L114 L229 | L160 L166 L177 L239 L315 L325 | L54 L81 L82 L83 L114 L204 | L132 L178 L315 L316 L325 | L55 L71 L82 L83 L208 L231 | L50 L63 L71 L74 L208 | A4 | L5 L21 L296 L346 | L7 L8 L14 L147 | A5 | L10 L174 L347 L349 | A6 | L11 L17 L24 L180 | L13 L16 L22 L113 | L15 L18 L266 L348 | A8 | A9 | A10 | L27 L31 L37 L102 | A11 | L28 L32 L104 L352 | L33 L75 L120 L359 | A12 | L39 L43 L117 L284 | A14 | L49 L92 L107 L256 | A15 | A16 | L68 L79 L138 L150 L205 | L68 L205 L279 L372 L376 L378 | L273 L285 L289 L368 L372 L378 | L273 L355 L358 L364 L368 L382 | L351 L357 L362 L364 L382 | A18 | A19 | L88 L97 L211 L249 | A22 | L108 L260 L283 L366 L375 L377 | L121 L291 L309 L371 L375 L377 | L234 L260 L268 L283 L290 | L215 L291 L371 L380 L381 L384 | L192 L354 L379 L380 L384 | L109 L134 L156 L272 L280 L287 | L109 L115 L148 L156 L161 L216 | L124 L139 L161 L216 L322 L335 | L165 L280 L287 L313 L334 | L190 L300 L318 L322 L335 | A23 | L127 L144 L149 L213 L221 L254 | L149 L254 L305 L310 L369 L370 | L136 L213 L221 L235 L294 L301 | L263 L302 L341 L369 L370 | L176 L281 L294 L301 L336 | A24 | A25 | A26 L163 | A26 L163 | L170 L343 L344 L350 | A27 | L173 A37 | L173 A37 | A28 | L186 A31 | L186 A31 | A30 | L199 L214 L219 L307 | A32 | A33 | A34 | A38 | A39 | A40 | A41 | A42 | A43 | L320 A48 | L320 A48 | A46 | A47 | A49 | A50 | A51 | A52 | A53
sketch "Skizze3" plane through (0, 1.5, 0) normal (0, 1, 0) x (-1, 0, 0)
  arc A0 (198, -200) -> (210, -188) centre (198, -188) ccw
  line L0 (210, -188) -> (210, 188)
  arc A1 (210, 188) -> (198, 200) centre (198, 188) ccw
  line L1 (198, 200) -> (-198, 200)
  arc A2 (-198, 200) -> (-210, 188) centre (-198, 188) ccw
  line L2 (-210, 188) -> (-210, -188)
  arc A3 (-210, -188) -> (-198, -200) centre (-198, -188) ccw
  line L3 (-198, -200) -> (198, -200)
  line L4 (0, -200) -> (0, 200)
  circle A4 centre (-168, 50.7) radius 1.6
  circle A5 centre (91.6, -62) radius 1.6
  line L5 (154.3, -57) -> (151.3, -57)
  line L6 (151.3, -57) -> (151.3, 13)
  line L7 (151.3, 13) -> (154.3, 13)
  line L8 (154.3, 13) -> (154.3, -57)
  line L9 (113.5, -57) -> (110.5, -57)
  line L10 (110.5, -57) -> (110.5, 13)
  line L11 (110.5, 13) -> (113.5, 13)
  line L12 (113.5, 13) -> (113.5, -57)
  line L13 (72.7, -57) -> (69.7, -57)
  line L14 (69.7, -57) -> (69.7, 13)
  line L15 (69.7, 13) -> (72.7, 13)
  line L16 (72.7, 13) -> (72.7, -57)
  line L17 (21.9, -57) -> (18.9, -57)
  line L18 (18.9, -57) -> (18.9, 13)
  line L19 (18.9, 13) -> (21.9, 13)
  line L20 (21.9, 13) -> (21.9, -57)
  circle A6 centre (0, -62) radius 1.6
  circle A7 centre (-40.8, -62) radius 1.6
  circle A8 centre (-132.4, -62) radius 1.6
  line L21 (-110.5, -57) -> (-113.5, -57)
  line L22 (-113.5, -57) -> (-113.5, 13)
  line L23 (-113.5, 13) -> (-110.5, 13)
  line L24 (-110.5, 13) -> (-110.5, -57)
  circle A9 centre (-91.6, 18) radius 1.6
  circle A10 centre (-168, 81.1) radius 1.6
  circle A11 centre (-56, 50.7) radius 1.6
  circle A12 centre (56, 81.1) radius 1.6
  circle A13 centre (166.5, 81.1) radius 1.6
  circle A14 centre (-56, -105) radius 1.6
  line L25 (-51, -135) -> (-51, -95)
  line L26 (-51, -95) -> (51, -95)
  line L27 (51, -95) -> (51, -135)
  line L28 (51, -135) -> (-51, -135)
  line L29 (61, -135) -> (61, -95)
  line L30 (61, -95) -> (163, -95)
  line L31 (163, -95) -> (163, -135)
  line L32 (163, -135) -> (61, -135)
  circle A15 centre (56, -125) radius 1.6
  line L33 (-61, -95) -> (-61, -135)
  line L34 (-61, -135) -> (-163, -135)
  line L35 (-163, -135) -> (-163, -95)
  line L36 (-163, -95) -> (-61, -95)
  circle A16 centre (166.5, 50.7) radius 1.6
  circle A17 centre (56, 50.7) radius 1.6
  circle A18 centre (-56, 81.1) radius 1.6
  circle A19 centre (-152.8, 18) radius 1.6
  circle A20 centre (-71.2, 18) radius 1.6
  line L37 (-130.9, 13) -> (-130.9, -57)
  line L38 (-130.9, -57) -> (-133.9, -57)
  line L39 (-133.9, -57) -> (-133.9, 13)
  line L40 (-133.9, 13) -> (-130.9, 13)
  circle A21 centre (-112, -62) radius 1.6
  line L41 (-39.3, -57) -> (-42.3, -57)
  line L42 (-42.3, -57) -> (-42.3, 13)
  line L43 (-42.3, 13) -> (-39.3, 13)
  line L44 (-39.3, 13) -> (-39.3, -57)
  line L45 (-1.5, 13) -> (1.5, 13)
  line L46 (1.5, 13) -> (1.5, -57)
  line L47 (1.5, -57) -> (-1.5, -57)
  line L48 (-1.5, -57) -> (-1.5, 13)
  line L49 (42.3, -57) -> (39.3, -57)
  line L50 (39.3, -57) -> (39.3, 13)
  line L51 (39.3, 13) -> (42.3, 13)
  line L52 (42.3, 13) -> (42.3, -57)
  line L53 (93.1, -57) -> (90.1, -57)
  line L54 (90.1, -57) -> (90.1, 13)
  line L55 (90.1, 13) -> (93.1, 13)
  line L56 (93.1, 13) -> (93.1, -57)
  line L57 (133.9, -57) -> (130.9, -57)
  line L58 (130.9, -57) -> (130.9, 13)
  line L59 (130.9, 13) -> (133.9, 13)
  line L60 (133.9, 13) -> (133.9, -57)
  circle A22 centre (152.8, -62) radius 1.6
  circle A23 centre (71.2, -62) radius 1.6
  circle A24 centre (-20.4, 18) radius 1.6
  circle A25 centre (20.4, -62) radius 1.6
  circle A26 centre (112, -62) radius 1.6
  circle A27 centre (152.8, 18) radius 1.6
  circle A28 centre (112, 18) radius 1.6
  circle A29 centre (71.2, 18) radius 1.6
  circle A30 centre (20.4, 18) radius 1.6
  circle A31 centre (-20.4, -62) radius 1.6
  circle A32 centre (-71.2, -62) radius 1.6
  circle A33 centre (-152.8, -62) radius 1.6
  line L61 (-93.1, -57) -> (-93.1, 13)
  line L62 (-93.1, 13) -> (-90.1, 13)
  line L63 (-90.1, 13) -> (-90.1, -57)
  line L64 (-90.1, -57) -> (-93.1, -57)
  circle A34 centre (-112, 18) radius 1.6
  line L65 (-61, 70.9) -> (-163, 70.9)
  line L66 (-163, 70.9) -> (-163, 91.3)
  line L67 (-163, 91.3) -> (-61, 91.3)
  line L68 (-61, 91.3) -> (-61, 70.9)
  line L69 (51, 40.5) -> (-51, 40.5)
  line L70 (-51, 40.5) -> (-51, 60.9)
  line L71 (-51, 60.9) -> (51, 60.9)
  line L72 (51, 60.9) -> (51, 40.5)
  line L73 (163, 91.3) -> (163, 70.9)
  line L74 (163, 70.9) -> (61, 70.9)
  line L75 (61, 70.9) -> (61, 91.3)
  line L76 (61, 91.3) -> (163, 91.3)
  circle A35 centre (-168, -105) radius 1.6
  circle A36 centre (-56, -125) radius 1.6
  circle A37 centre (166.5, -125) radius 1.6
  circle A38 centre (166.5, -105) radius 1.6
  circle A39 centre (56, -105) radius 1.6
  circle A40 centre (-168, -125) radius 1.6
  line L77 (163, 60.9) -> (163, 40.5)
  line L78 (163, 40.5) -> (61, 40.5)
  line L79 (61, 40.5) -> (61, 60.9)
  line L80 (61, 60.9) -> (163, 60.9)
  line L81 (51, 91.3) -> (51, 70.9)
  line L82 (51, 70.9) -> (-51, 70.9)
  line L83 (-51, 70.9) -> (-51, 91.3)
  line L84 (-51, 91.3) -> (51, 91.3)
  line L85 (-61, 60.9) -> (-61, 40.5)
  line L86 (-61, 40.5) -> (-163, 40.5)
  line L87 (-163, 40.5) -> (-163, 60.9)
  line L88 (-163, 60.9) -> (-61, 60.9)
  circle A41 centre (-132.4, 18) radius 1.6
  line L89 (-72.7, 13) -> (-69.7, 13)
  line L90 (-69.7, 13) -> (-69.7, -57)
  line L91 (-69.7, -57) -> (-72.7, -57)
  line L92 (-72.7, -57) -> (-72.7, 13)
  line L93 (-151.3, 13) -> (-151.3, -57)
  line L94 (-151.3, -57) -> (-154.3, -57)
  line L95 (-154.3, -57) -> (-154.3, 13)
  line L96 (-154.3, 13) -> (-151.3, 13)
  circle A42 centre (-91.6, -62) radius 1.6
  line L97 (-18.9, -57) -> (-21.9, -57)
  line L98 (-21.9, -57) -> (-21.9, 13)
  line L99 (-21.9, 13) -> (-18.9, 13)
  line L100 (-18.9, 13) -> (-18.9, -57)
  circle A43 centre (0, 18) radius 1.6
  circle A44 centre (40.8, 18) radius 1.6
  circle A45 centre (91.6, 18) radius 1.6
  circle A46 centre (132.4, 18) radius 1.6
  circle A47 centre (132.4, -62) radius 1.6
  circle A48 centre (40.8, -62) radius 1.6
  circle A49 centre (-40.8, 18) radius 1.6
  point P0 (100, -180)
  point P1 (190, 115)
  point P2 (190, -80)
  point P3 (100, 175)
  point P4 (-100, 175)
  point P5 (-190, 115)
  point P6 (-190, -80)
  point P7 (-100, -180)
  dimension "d60" = 60
  dimension "d61" = 100
  dimension "d62" = 100
  dimension "d63" = 20
  dimension "d64" = 195
  dimension "d65" = 100
  dimension "d66" = 90
  dimension "d67" = 90
  constraint midpoint L3 L4.start
  constraint midpoint L1 L4.end
  constraint symmetric P0 L4 P7
  constraint symmetric P1 L4 P5
  constraint symmetric P2 L4 P6
  constraint symmetric P3 L4 P4
  measures "d60" vertical distance of P1 P3
  measures "d61" vertical distance of P0 P2
  measures "d62" horizontal distance of P0 L4.start
  measures "d63" distance of L3 P0
  measures "d64" distance of P1 P2
  measures "d65" distance of P3 L4
  measures "d66" horizontal distance of P0 P2
  measures "d67" horizontal distance of P1 P3
hole "Bohrung1" at (-190, 1.5, 115) at (-100, 1.5, 175) at (100, 1.5, 175) at (190, 1.5, 115) at (190, 1.5, -80) at (100, 1.5, -180) at (-100, 1.5, -180) at (-190, 1.5, -80) direction (0, -1, 0) diameter 3.2 depth 70 tip angle 118
